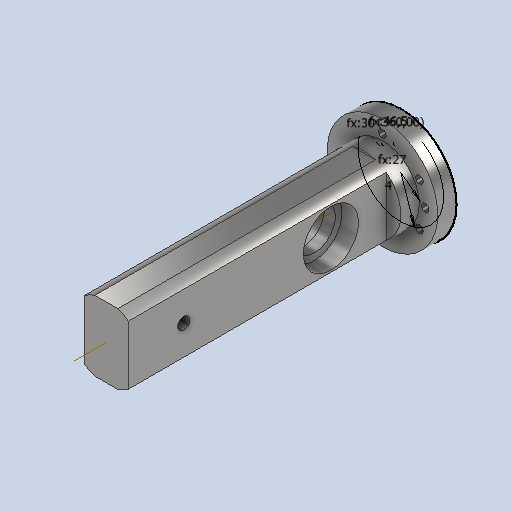
# Autodesk Inventor part: Flansch_FemalePart_MainAxis_HeadConnectorBase
Saved by Autodesk Inventor 2022 (Build 260153000, 153)
## iProperties
Created: 2022-07-15
Part Number: Flansch_FemalePart_MainAxis_HeadConnectorBase
Material: Edelstahl
Document SubType Name: Modeling
Designer: alexw
Density: 8 g/cm^3
Appearance: Halbpoliert
Mass: 1180.63 g
Surface Area: 277.802 cm^2
Volume: 147.578 cm^3
Flansch_ParralelMech_FlatPart_Width: 140,000 mm
Total_Bearing_Hole_Dist: 80,000 mm
MainAxis_Schluesselweite: 24,000 mm
Author: alexw
Autodesk Inventor part; units mm, degrees
ref_plane "YZ Plane" through (0, 0, 0) normal (1, 0, 0) x (0, 1, 0)
ref_plane "XZ Plane" through (0, 0, 0) normal (0, 1, 0) x (-1, 0, 0)
ref_plane "XY Plane" through (0, 0, 0) normal (0, 0, 1) x (1, 0, 0)
sketch "Skizze1" plane through (0, 0, 0) normal (0, 0, 1) x (1, 0, 0)
  circle A0 centre (0, 0) radius 30
  circle A1 centre (0, 0) radius 13.5
  circle A2 centre (0, 0) radius 9.5
  circle A3 centre (0, 0) radius 23.25 construction
  line L0 (0, 0) -> (0, 23.25) construction
  point P0 (-23.25, 0)
  point P1 (0, -23.25)
  point P2 (23.25, 0)
  dimension "d4" = 46.5
  dimension "d0" = 4
  dimension "d1" = 27
  dimension "d3" = 30
  dimension "d7" = 360
  constraints: 4 coincident, 3 centre point, 2 end point, 1 vertical, 1 vertical alignment, 7 other
  measures "d0" radial gap between concentric circles of A2 A1
  measures "d1" diameter of A1
  measures "d3" radius of A0
extrude "Extrusion1" add sketch "Skizze1" along normal blind 10 contours A0 | A1
extrude "Extrusion2" add sketch "Skizze1" against normal blind 2.6 contours A1
sketch "Skizze2" plane through (0, 0, 10) normal (0, 0, 1) x (1, 0, 0)
  point P0 (0, 0)
  point P1 (0, 23.25)
  point P2 (20.1351, 11.625)
  point P3 (20.1351, -11.625)
  point P4 (23.25, 0)
  point P5 (0, -23.25)
  point P6 (-23.25, 0)
hole "Bohrung1" at (0, 23.25, 10) at (20.1351, 11.625, 10) at (20.1351, -11.625, 10) at (23.25, 0, 10) at (0, -23.25, 10) at (-23.25, 0, 10) direction (0, 0, -1) diameter 4.134 end through all thread size "M5x0.8" class "6H" standard "ISO Metric profile"
ref_plane "Arbeitsebene1" through (0, 0, 10) normal (0, 0, 1) x (1, 0, 0)
sketch "Skizze4" plane through (0, 0, 0) normal (1, 0, 0) x (0, 1, 0)
  line L0 (9.5, -2.6) -> (-9.5, -2.6) construction
  line L1 (0, 192.52) -> (0, -35.12) construction
  line L2 (-9.5, 10) -> (-9.5, -2.6) construction
  line L3 (9.5, 10) -> (9.5, -2.6) construction
  line L4 (-9.5, 10) -> (9.5, 10) construction
  line L5 (-9.5, 2.4) -> (9.5, 2.4)
  line L6 (-9.5, 2.4) -> (-9.5, 10)
  line L7 (-9.5, 10) -> (-20, 10)
  line L8 (-20, 10) -> (-20, 160)
  line L9 (-20, 160) -> (20, 160)
  line L10 (20, 10) -> (9.5, 10)
  line L11 (9.5, 10) -> (9.5, 2.4)
  line L12 (20, 160) -> (20, 10)
  line L13 (0, 2.4) -> (0, 160)
  point P0 (0, 0)
  dimension "d27" = 5
  dimension "d31" = 150
  dimension "d33" = 40
  constraints: 18 end point, 5 point on line, 3 perpendicular, 2 collinear, 2 midpoint, 1 horizontal, 1 vertical
  measures "d27" distance between parallel lines of L5 L0
  measures "d31" distance between parallel lines of L7 L9
  measures "d33" distance between parallel lines of L12 L8
revolve "Umdrehung1" add sketch "Skizze4" angle 360 about axis through (0, 0, 0) along (0, 0, -1) contours L13 L9 L12 L10 L11 L5
sketch "Skizze5" plane through (0, 0, 160) normal (0, 0, 1) x (1, 0, 0)
  circle A0 centre (0, 0) radius 20
  line L0 (-12, 16) -> (-12, -16)
  line L1 (12, 16) -> (12, -16)
  line L2 (-6.245, 19) -> (6.245, 19)
  circle A1 centre (0, 0) radius 20 construction
  dimension "MainAxis_Schluesselweite" = 24
  dimension "d46" = 1
  dimension "d52" = 32
  constraints: 6 end point, 6 point on circle, 2 concentric, 2 vertical, 1 centre point, 1 horizontal, 1 parallel
  measures "MainAxis_Schluesselweite" distance between parallel lines of L1 L0
  measures "d46" distance edge to line of A0 L2
  measures "d52" distance of L0.start L0.end
extrude "Extrusion3" cut sketch "Skizze5" against normal blind 140 contours A0 L1 | A0 L0
sketch "Skizze6" plane through (0, 0, 0) normal (1, 0, 0) x (0, 1, 0)
  line L0 (-16, 160) -> (16, 160) construction
  line L1 (-16, 20) -> (16, 20) construction
  line L2 (0, -32) -> (0, 192) construction
  line L3 (-16, 20) -> (-16, 160) projected
  line L4 (16, 160) -> (16, 20) projected
  point P0 (0, 0)
  dimension "Flansch_ParralelMech_FlatPart_Width" = 140
  measures "Flansch_ParralelMech_FlatPart_Width" distance between parallel lines of L0 L1
ref_plane "Arbeitsebene2" through (0, 0, 90) normal (0, 0, 1) x (1, 0, 0)
ref_plane "Arbeitsebene3" through (0, 0, 50) normal (0, 0, 1) x (1, 0, 0)
ref_plane "Arbeitsebene4" through (0, 0, 130) normal (0, 0, 1) x (1, 0, 0)
extrude "Extrusion4" cut sketch "Skizze5" against normal blind 140 contours L2 A0
sketch "Skizze7" plane through (0, 0, 50) normal (0, 0, 1) x (1, 0, 0)
  line L0 (-12, 16) -> (-12, -16) construction
  line L1 (-12, 15) -> (-3, 15)
  line L2 (-3, 15) -> (-3, 11.425)
  line L3 (-3, 11.425) -> (3, 11.425)
  line L4 (3, 11.425) -> (3, 15)
  line L5 (3, 15) -> (12, 15)
  line L6 (-12, 0) -> (-12, 15)
  line L7 (0, -16) -> (0, 16) construction
  line L8 (12, -16) -> (12, 16) construction
  line L9 (12, 15) -> (12, 0)
  line L10 (-12, 0) -> (12, 0)
  line L11 (-42, 0) -> (42, 0) construction
  point P0 (0, 11.425)
  point P1 (-12, -7.2111)
  point P2 (12, 7.2111)
  dimension "d51" = 9
  dimension "d63" = 30
  dimension "d64" = 22.85
  constraints: 16 end point, 5 point on line, 4 perpendicular, 3 midpoint, 1 horizontal, 1 vertical
  measures "d51" distance between parallel lines of L0 L2
  measures "d63" diameter of L1 L10
  measures "d64" diameter of L3 L10
revolve "Umdrehung2" cut sketch "Skizze7" angle 360 about axis through (-10, 0, 50) along (1, 0, 0)
ref_plane "Arbeitsebene5" through (0, 0, 85) normal (1, 0, 0) x (0, 0, -1)
sketch "Skizze8" plane through (12, -16, 160) normal (1, 0, 0) x (0, 0, -1)
  line L0 (30, -26) -> (30, 58) construction
  line L1 (-32.52, 16) -> (195.12, 16) construction
  point P0 (160, 16)
  point P1 (30, 16)
  constraints: 1 midpoint, 1 point on line
hole "Bohrung2" at (12, 0, 130) direction (-1, 0, 0) diameter 6.647 end through all thread size "M8x1.25" class "6H" standard "ISO Metric profile"
mirror "Spiegeln2" about plane through (0, 0, 0) normal (0, 1, 0) of "Extrusion4"
equation "\"d4\" = Flansch_FemalePart_HoleDia"
equation "\"d1\" = Flansch_Klemmdeckelausnahme_Dia"
equation "\"d3\" = Flansch_FemalePart_OuterDia"
equation "\"d33\" = d28"
equation "\"d47\" = Flansch_ParralelMech_FlatPart_Width"
equation "\"Total_Bearing_Hole_Dist\" = 80"
equation "\"Flansch_FemalePart_HoleDia\" = 46.5"
equation "\"Flansch_Klemmdeckelausnahme_Dia\" = 27"
equation "\"Flansch_FemalePart_OuterDia\" = 30"
equation "\"d28\" = 40"
